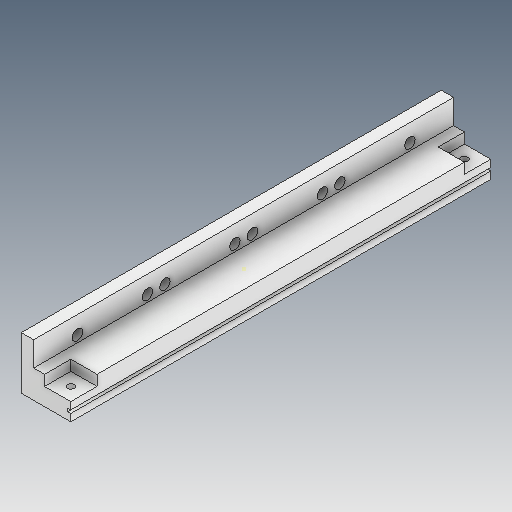
# Autodesk Inventor part: horizontal_Edge
Saved by Autodesk Inventor 2027 (Build 310192060, 192F)
## iProperties
Created: 2026-07-26
Part Number: horizontal_Edge
Material: ABS Plastic
Document SubType Name: Modeling
Designer: prest
Density: 1.06 g/cm^3
Appearance: Smooth - White
Author: prest
Autodesk Inventor part; units mm, degrees
ref_plane "YZ Plane" through (0, 0, 0) normal (1, 0, 0) x (0, 1, 0)
ref_plane "XZ Plane" through (0, 0, 0) normal (0, 1, 0) x (-1, 0, 0)
ref_plane "XY Plane" through (0, 0, 0) normal (0, 0, 1) x (1, 0, 0)
sketch "Sketch1" plane through (0, 0, 0) normal (0, 1, 0) x (-1, 0, 0)
  line L0 (15, 120) -> (-15, 120)
  line L1 (-15, 120) -> (-15, -120)
  line L2 (-15, -120) -> (15, -120)
  line L3 (15, -120) -> (15, 120)
  point P0 (0, 0)
  point P1 (0, 120)
  point P2 (15, 0)
  dimension "d0" = 240
  dimension "d1" = 30
  constraints: 8 end point, 2 midpoint, 2 parallel, 1 horizontal, 1 horizontal alignment, 1 perpendicular, 1 vertical alignment
  measures "d0" distance of L2.end L0.start
  measures "d1" distance of L0.start L0.end
extrude "Extrusion1" add sketch "Sketch1" along normal blind 15
sketch "Sketch2" plane through (0, 15, 0) normal (0, 1, 0) x (1, 0, 0)
  line L0 (-15, 120) -> (-15, -120) projected
  line L1 (15, 120) -> (-15, 120) projected
  line L2 (-15, -120) -> (-5, -120)
  line L3 (-5, -120) -> (-5, 120)
  line L4 (-5, 120) -> (-15, 120)
  line L5 (-15, 120) -> (-15, -120)
  point P0 (0, 0)
  dimension "d4" = 10
  constraints: 8 end point, 2 parallel, 1 horizontal, 1 perpendicular, 1 point on line
  measures "d4" distance of L0.end L2.end
extrude "Extrusion2" add sketch "Sketch2" along normal blind 10
sketch "Sketch4" plane through (0, 15, 0) normal (0, 1, 0) x (1, 0, 0)
  line L0 (15, 120) -> (-5, 120) projected
  line L1 (15, -120) -> (15, 120) projected
  line L2 (15, -120) -> (0, -120)
  line L3 (0, -120) -> (0, -105)
  line L4 (0, -105) -> (15, -105)
  line L5 (15, -105) -> (15, -120)
  point P0 (0, 0)
  dimension "d42" = 15
  dimension "d43" = 15
  constraints: 8 end point, 2 parallel, 1 horizontal, 1 perpendicular
  measures "d42" distance of L2.end L3.end
  measures "d43" distance of L3.end L4.end
extrude "Extrusion3" cut sketch "Sketch4" against normal blind 10
sketch "Sketch5" plane through (0, 5, 0) normal (0, 1, 0) x (1, 0, 0)
  line L0 (15, -120) -> (15, 120) projected
  line L1 (0, -105) -> (15, -105) projected
  line L2 (15, -120) -> (0, -105) construction
  line L3 (-15, -120) -> (15, -120) projected
  line L4 (0, -120) -> (15, -105) construction
  point P0 (0, 0)
  point P1 (7.5, -112.5)
  point P2 (7.5, -112.5)
  constraints: 4 end point, 1 coincident, 1 midpoint
hole "Hole2" at (7.5, 5, 112.5) direction (0, -1, 0) diameter 4 depth 4
mirror "Mirror1" about plane through (0, 0, 0) normal (0, 0, 1) of "Extrusion3", "Hole2"
move faces "Move1" translate (0, -5, 0) faces at (5, 0, 40)
move faces "Move3" translate (1.716, 0, 0) faces at (-15, 5, -40)
move faces "Move4" translate (-1.213, 0, 0) faces at (-5, 18.3333, 40)
move faces "Move5" translate (0, -4, 0) faces at (10, 15, 35)
sketch "Sketch6" plane through (-6.213, 25, 120) normal (1, 0, 0) x (0, 0, -1)
  point P0 (120, -25)
sketch "Sketch7" plane through (-6.213, 25, 120) normal (1, 0, 0) x (0, 0, -1)
  line L0 (0, 0) -> (240, 0) projected
  line L1 (225, -14) -> (240, -14) projected
  line L2 (0, -14) -> (0, 0) projected
  line L3 (0, -30) -> (0, 0) projected
  line L4 (240, -30) -> (240, 0) projected
  point P0 (120, -25)
  point P1 (215, -10)
  point P2 (175, -10)
  point P3 (165, -10)
  point P4 (125, -10)
  point P5 (115, -10)
  point P6 (75, -10)
  point P7 (65, -10)
  point P8 (0, -7)
  point P9 (25, -10)
  dimension "d82" = 40
  dimension "d83" = 10
  dimension "d84" = 40
  dimension "d85" = 10
  dimension "d86" = 40
  dimension "d87" = 10
  dimension "d91" = 10
  dimension "d93" = 40
  dimension "d96" = 25
  constraints: 7 horizontal alignment, 1 midpoint
  measures "d82" distance of point (175, -10) point (215, -10)
  measures "d83" distance of point (165, -10) point (175, -10)
  measures "d84" distance of point (125, -10) point (165, -10)
  measures "d85" distance of point (115, -10) point (125, -10)
  measures "d86" distance of point (75, -10) point (115, -10)
  measures "d87" distance of point (65, -10) point (75, -10)
  measures "d91" distance from line of L0 point (215, -10)
  measures "d93" distance of point (65, -10) point (25, -10)
  measures "d96" distance from line of L4 point (215, -10)
hole "Hole3" at (-6.213, 15, 55) at (-6.213, 15, 45) at (-6.213, 15, 5) at (-6.213, 15, -5) at (-6.213, 15, -45) at (-6.213, 15, -55) at (-6.213, 15, -95) at (-6.213, 15, 95) direction (-1, 0, 0) diameter 6 end through all
sketch "Sketch8" plane through (15, 5, 120) normal (1, 0, 0) x (0, 0, -1)
  line L0 (240, -10) -> (240, 20) projected
  line L1 (0, -10) -> (0, 20) projected
  line L2 (240, -10) -> (240, 0) projected
  line L3 (203.8731, -5) -> (-4.7144, -5)
  line L4 (240, -5.9) -> (0, -5.9)
  line L5 (240, -4.1) -> (0, -4.1)
  line L6 (240, -4.1) -> (240, -5.9)
  line L7 (0, -4.1) -> (0, -5.9)
  point P0 (120, -5)
  point P1 (240, -5)
  point P2 (99.5794, -5)
  point P3 (240, -5)
  point P4 (0, -4.1)
  dimension "d78" = 1.8
  constraints: 10 end point, 3 midpoint, 2 perpendicular, 2 point on line, 2 symmetric about line, 1 collinear, 1 horizontal, 1 horizontal alignment
  measures "d78" diameter of L4 L3
extrude "Extrusion4" cut sketch "Sketch8" against normal blind 1.8
equation "\"d84\" = d82"
equation "\"d85\" = d83"
equation "\"d86\" = d84"
equation "\"d87\" = d85"
equation "\"d93\" = d82"
body "Solid1"
